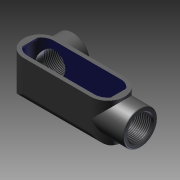
# Autodesk Inventor part: L37-TB
Saved by Autodesk Inventor 2015 (Build 190159000, 159)
## iProperties
Category: PARTsolutions
Company: THOMASBETTS
Created: 2015-01-24
Part Number: L37-TB
Catalog Web Link: www.cadenas.de
Description: L Form 7 BlueKote-Conduit Bodies
Vendor: THOMASBETTS
Document SubType Name: Modeling
Designer: PARTuser1
Manufacturer: THOMASBETTS
Mass: 103.745 g
Surface Area: 413.869 cm^2
Volume: 103.745 cm^3
Density: 1 g/cm^3
Material: Generic
Appearance: PSOLRGB-175-175-175
PSOL_IDENT_0: {$CADENAS_DATA\23d-libs\thomas_betts\fittings\conduit_outlet_bodies\l_form_7_bcb.prj},165 {VTYP=3D},
PSOL_IDENT_1: {NB=L37-TB},{LINA=L37-TB},{NN=L Form 7 BlueKote},{DATE=18.06.2010 06:16:34},{GEOMDATE=18.06.2010 06:
PSOL_IDENT_2: 15:00},{VERSION=},{LINEID=30},{LINESUBID=-1},{WBVAR=}  {NB=L37-TB},{LINA=L37-TB},{KT=DUMMY},{CN=L37-
PSOL_IDENT_3: TB},{HS=1.00000000},{A=6.020},{B=2.000},{C=2.562},{C2=1.687},{C3=1.750},{D=1.350},{E=4.550},{E2=0.32
PSOL_IDENT_4: 7},{CI=10.6},{BL=5.204},{BH=2.000},{BW=1.750},{BR1=0.875},{BR2=0.675},{LL=4.550},{LW=0.792},{MT=0.20
PSOL_IDENT_5: },{LBH=3.456},{HSH=1.673},{HL1=0.940},{HL2=0.780},{HH1=1.750},{HH2=1.155},{HH3=1.21},{HR1=0.150},{HR
PSOL_IDENT_6: 2=0.080},{HR3=0.080},{NDM=1.31500}
SUPPLIER: THOMASBETTS
ARTICLENO: L37-TB
BOMINFO: L37-TB
CREATOR: CADENAS GmbH
Title: L37-TB
Author: Cadenas PARTsolutions
Comments: Conduit Bodies
Autodesk Inventor part; units mm, degrees
ref_plane "YZ Plane" through (0, 0, 0) normal (1, 0, 0) x (0, 1, 0)
ref_plane "XZ Plane" through (0, 0, 0) normal (0, 1, 0) x (-1, 0, 0)
ref_plane "XY Plane" through (0, 0, 0) normal (0, 0, 1) x (1, 0, 0)
sketch "Sketch_1" plane through (0, 0, 0) normal (1, 0, 0) x (0, 1, 0)
  line L0 (50.8, 22.225) -> (10.16, 22.225)
  arc A0 (10.16, 22.225) -> (0, 12.065) centre (10.16, 12.065) ccw
  line L1 (0, 12.065) -> (0, -12.065)
  arc A1 (0, -12.065) -> (10.16, -22.225) centre (10.16, -12.065) ccw
  line L2 (10.16, -22.225) -> (50.8, -22.225)
  line L3 (50.8, -22.225) -> (50.8, 22.225)
  constraints: 8 end point, 4 point on circle, 2 centre point
extrude "Extrusion1" add sketch "Sketch_1" along normal mid plane 132.1816
sketch "Sketch_10" plane through (0, 0, 0) normal (0, 1, 0) x (-1, 0, 0)
  circle A0 centre (0, 0) radius 132.1816
  arc A1 (43.8658, -22.225) -> (43.8658, 22.225) centre (43.8658, 0) ccw
  line L0 (43.8658, 22.225) -> (-43.8658, 22.225)
  arc A2 (-43.8658, 22.225) -> (-43.8658, -22.225) centre (-43.8658, 0) ccw
  line L1 (-43.8658, -22.225) -> (43.8658, -22.225)
  constraints: 4 end point, 4 point on circle, 3 centre point
extrude "Extrusion2" cut sketch "Sketch_10" along normal blind 50.8
sketch "Sketch_7" plane through (0, 0, 0) normal (0, 0, 1) x (1, 0, 0)
  line L0 (86.8172, 25.4) -> (10.3632, 25.4)
  line L1 (10.3632, 25.4) -> (10.3632, 46.1433)
  arc A0 (11.8449, 47.625) -> (10.3632, 46.1433) centre (11.8449, 46.1433) ccw
  line L2 (11.8449, 47.625) -> (85.3355, 47.625)
  arc A1 (86.8172, 46.1433) -> (85.3355, 47.625) centre (85.3355, 46.1433) ccw
  line L3 (86.8172, 46.1433) -> (86.8172, 25.4)
  line L4 (86.8172, 25.4) -> (10.3632, 25.4)
  constraints: 10 end point, 4 point on circle, 2 centre point
revolve "Revolution1" add sketch "Sketch_7" angle 360 about axis through (86.8172, 25.4, 0) along (1, 0, 0)
sketch "Sketch_14" plane through (-43.8658, 0, 0) normal (1, 0, 0) x (0, 0, -1)
  line L0 (42.8498, 25.4) -> (0, 25.4)
  line L1 (0, 25.4) -> (0, 47.625)
  line L2 (0, 47.625) -> (41.3681, 47.625)
  arc A0 (42.8498, 46.1433) -> (41.3681, 47.625) centre (41.3681, 46.1433) ccw
  line L3 (42.8498, 46.1433) -> (42.8498, 25.4)
  line L4 (42.8498, 25.4) -> (0, 25.4)
  constraints: 10 end point, 2 point on circle, 1 centre point
revolve "Revolution2" add sketch "Sketch_14" angle 360 about axis through (-43.8658, 25.4, -42.8498) along (0, 0, -1)
sketch "Sketch_15" plane through (0, 0, 0) normal (1, 0, 0) x (0, 1, 0)
  line L0 (50.8, 17.145) -> (0, 17.145)
  arc A0 (0, 17.145) -> (-7.62, 9.525) centre (0, 9.525) ccw
  line L1 (-7.62, 9.525) -> (-7.62, -9.525)
  arc A1 (-7.62, -9.525) -> (0, -17.145) centre (0, -9.525) ccw
  line L2 (0, -17.145) -> (50.8, -17.145)
  line L3 (50.8, -17.145) -> (50.8, 17.145)
  constraints: 8 end point, 4 point on circle, 2 centre point
sketch "Sketch_17" plane through (0, 0, 0) normal (0, 0, 1) x (1, 0, 0)
  line L0 (-43.8912, -7.62) -> (-43.8912, 50.8)
  line L1 (-43.8912, 50.8) -> (-26.7462, 50.8)
  line L2 (-26.7462, 50.8) -> (-26.7462, 0)
  arc A0 (-34.3662, -7.62) -> (-26.7462, 0) centre (-34.3662, 0) ccw
  line L3 (-34.3662, -7.62) -> (-43.8912, -7.62)
  line L4 (-43.8912, -7.62) -> (-43.8912, 50.8)
  constraints: 10 end point, 2 point on circle, 1 centre point
revolve "Revolution3" cut sketch "Sketch_17" angle 360 about axis through (-43.8912, -7.62, 0) along (0, -1, 0)
extrude "Extrusion3" cut sketch "Sketch_15" along normal mid plane 87.7824
sketch "Sketch_3" plane through (0, 0, 0) normal (0, 0, 1) x (1, 0, 0)
  line L0 (43.8912, -7.62) -> (43.8912, 50.8)
  line L1 (43.8912, 50.8) -> (61.0362, 50.8)
  line L2 (61.0362, 50.8) -> (61.0362, 0)
  arc A0 (53.4162, -7.62) -> (61.0362, 0) centre (53.4162, 0) ccw
  line L3 (53.4162, -7.62) -> (43.8912, -7.62)
  line L4 (43.8912, -7.62) -> (43.8912, 50.8)
  constraints: 10 end point, 2 point on circle, 1 centre point
revolve "Revolution4" cut sketch "Sketch_3" angle 360 about axis through (43.8912, -7.62, 0) along (0, -1, 0)
sketch "Sketch_8" plane through (0, 50.8, 0) normal (0, 1, 0) x (1, 0, 0)
  arc A0 (57.785, -13.9449) -> (57.785, 13.9449) centre (43.8912, 0) ccw
  line L0 (57.785, 13.9449) -> (57.785, -13.9449)
  constraints: 2 end point, 2 point on circle, 1 centre point
extrude "Extrusion4" add sketch "Sketch_8" against normal blind 2.54
sketch "Sketch_9" plane through (0, 50.8, 0) normal (0, 1, 0) x (1, 0, 0)
  arc A0 (-57.785, 13.9449) -> (-57.785, -13.9449) centre (-43.8912, 0) ccw
  line L0 (-57.785, -13.9449) -> (-57.785, 13.9449)
  constraints: 2 end point, 2 point on circle, 1 centre point
extrude "Extrusion5" add sketch "Sketch_9" against normal blind 2.54
sketch "Sketch_4" plane through (0, 0, 0) normal (0, 1, 0) x (-1, 0, 0)
  arc A0 (-57.785, 13.9449) -> (-57.785, -13.9449) centre (-43.8912, 0) ccw
  line L0 (-57.785, -13.9449) -> (-57.785, 13.9449)
  constraints: 2 end point, 2 point on circle, 1 centre point
extrude "Extrusion6" add sketch "Sketch_4" along normal blind 2.54
sketch "Sketch_5" plane through (0, 0, 0) normal (0, 1, 0) x (-1, 0, 0)
  arc A0 (57.785, -13.9449) -> (57.785, 13.9449) centre (43.8912, 0) ccw
  line L0 (57.785, 13.9449) -> (57.785, -13.9449)
  constraints: 2 end point, 2 point on circle, 1 centre point
extrude "Extrusion7" add sketch "Sketch_5" along normal blind 2.54
sketch "Sketch_6" plane through (0, 0, 0) normal (1, 0, 0) x (0, 1, 0)
  line L0 (2.54, 22.225) -> (-50.8, 22.225)
  line L1 (-50.8, 22.225) -> (-50.8, -22.225)
  line L2 (-50.8, -22.225) -> (2.54, -22.225)
  line L3 (2.54, -22.225) -> (2.54, -18.7852)
  arc A0 (0, -12.065) -> (2.54, -18.7852) centre (10.16, -12.065) ccw
  line L4 (0, -12.065) -> (0, 12.065)
  arc A1 (2.54, 18.7852) -> (0, 12.065) centre (10.16, 12.065) ccw
  line L5 (2.54, 18.7852) -> (2.54, 22.225)
  constraints: 12 end point, 4 point on circle, 2 centre point
extrude "Extrusion8" cut sketch "Sketch_6" along normal mid plane 132.1816
sketch "Sketch_11" plane through (0, 0, 0) normal (0, 0, 1) x (1, 0, 0)
  line L0 (86.8172, 25.4) -> (10.3632, 25.4)
  line L1 (10.3632, 25.4) -> (10.3632, 38.9999)
  line L2 (10.3632, 38.9999) -> (85.3511, 41.341)
  line L3 (85.3511, 41.341) -> (86.8172, 42.8536)
  line L4 (86.8172, 42.8536) -> (86.8172, 25.4)
  line L5 (86.8172, 25.4) -> (10.3632, 25.4)
  constraints: 12 end point
revolve "Revolution5" cut sketch "Sketch_11" angle 360 about axis through (86.8172, 25.4, 0) along (1, 0, 0)
thread "Thread1" size "1" designation "1 - 11.5 NPT" standard "NPT" length 23.876 offset 10.5764
sketch "Sketch_12" plane through (-43.8658, 0, 0) normal (1, 0, 0) x (0, 0, -1)
  line L0 (42.8498, 25.4) -> (0, 25.4)
  line L1 (0, 25.4) -> (0, 40.049)
  line L2 (0, 40.049) -> (41.3837, 41.341)
  line L3 (41.3837, 41.341) -> (42.8498, 42.8536)
  line L4 (42.8498, 42.8536) -> (42.8498, 25.4)
  line L5 (42.8498, 25.4) -> (0, 25.4)
  constraints: 12 end point
revolve "Revolution6" cut sketch "Sketch_12" angle 360 about axis through (-43.8658, 25.4, -42.8498) along (0, 0, -1)
thread "Thread2" size "1" designation "1 - 11.5 NPT" standard "NPT" length 22.4208
body "Solid1"
